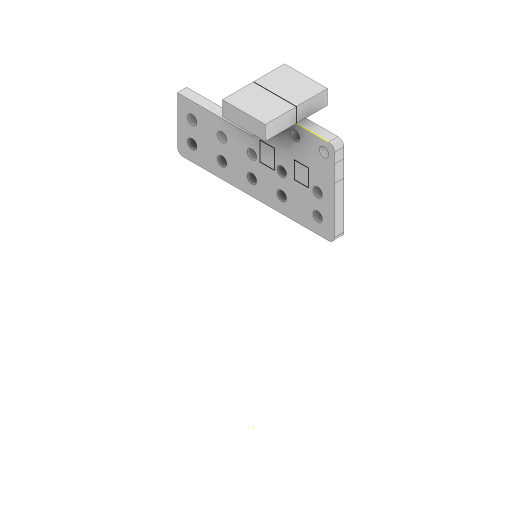
# Autodesk Inventor part: upper diod hplder
Saved by Autodesk Inventor 2023.2 (Build 272271000, 271)
## iProperties
Created: 2023-04-12
Part Number: upper diod hplder
Material: Типовые
Document SubType Name: Modeling
Designer: User
Density: 1 g/cm^3
Appearance: По умолчанию
Author: User
Autodesk Inventor part; units mm, degrees
(part 1 of 6)
ref_plane "YZ Plane" through (0, 0, 0) normal (1, 0, 0) x (0, 1, 0)
ref_plane "XZ Plane" through (0, 0, 0) normal (0, 1, 0) x (-1, 0, 0)
ref_plane "XY Plane" through (0, 0, 0) normal (0, 0, 1) x (1, 0, 0)
sketch "Эскиз1" plane through (0, 0, 0) normal (0, 0, 1) x (1, 0, 0)
  line L0 (-26.3398, -17.2609) -> (28.1261, -17.2901)
  arc A0 (28.1261, -17.2901) -> (29.0872, -16.3296) centre (28.1266, -16.3296) ccw
  line L1 (29.0872, -16.3296) -> (29.0872, 55.0102)
  arc A1 (29.0872, 55.0102) -> (28.1266, 55.9707) centre (28.1266, 55.0102) ccw
  line L2 (28.1266, 55.9707) -> (-6.6805, 55.9707)
  line L3 (-6.6805, 55.9707) -> (-6.6805, 56.9313)
  line L4 (-6.6805, 56.9313) -> (28.1266, 56.9313)
  arc A2 (30.0477, 55.0102) -> (28.1266, 56.9313) centre (28.1266, 55.0102) ccw
  line L5 (30.0477, 55.0102) -> (30.0477, -16.3296)
  arc A3 (28.1256, -18.2506) -> (30.0477, -16.3296) centre (28.1266, -16.3296) ccw
  line L6 (28.1256, -18.2506) -> (-26.3547, -18.2215)
  arc A4 (-28.2747, -16.2994) -> (-26.3547, -18.2215) centre (-26.3537, -16.3004) ccw
  line L7 (-28.2747, -16.2994) -> (-28.2581, 14.7062)
  line L8 (-28.2581, 14.7062) -> (-28.2581, 55.0102)
  arc A5 (-26.3371, 56.9313) -> (-28.2581, 55.0102) centre (-26.3371, 55.0102) ccw
  line L9 (-26.3371, 56.9313) -> (-24.7345, 56.9313)
  line L10 (-24.7345, 56.9313) -> (-24.7345, 55.9729)
  line L11 (-24.7345, 55.9729) -> (-26.3371, 55.9729)
  arc A6 (-26.3371, 55.9729) -> (-27.2998, 55.0102) centre (-26.3371, 55.0102) ccw
  line L12 (-27.2998, 55.0102) -> (-27.2998, -16.3004)
  arc A7 (-27.2998, -16.3004) -> (-26.3398, -17.2609) centre (-26.3393, -16.3004) ccw
  line L13 (-24.4159, 86.3863) -> (-24.4159, 89.6301)
  arc A8 (-22.4948, 91.5512) -> (-24.4159, 89.6301) centre (-22.4948, 89.6301) ccw
  line L14 (-22.4948, 91.5512) -> (24.2451, 91.5512)
  arc A9 (26.1661, 89.6301) -> (24.2451, 91.5512) centre (24.2451, 89.6301) ccw
  line L15 (26.1661, 89.6301) -> (26.1661, 86.3863)
  arc A10 (-24.4154, 65.9583) -> (-22.4943, 64.0372) centre (-22.4943, 65.9583) ccw
  line L16 (-24.4154, 65.9583) -> (-24.4154, 80.9805)
  line L17 (26.1662, 80.9805) -> (26.1662, 65.9583)
  arc A11 (24.2452, 64.0372) -> (26.1662, 65.9583) centre (24.2452, 65.9583) ccw
  line L18 (24.2452, 64.0372) -> (-22.4943, 64.0372)
  line L19 (22.2378, -70.3584) -> (22.2378, -67.7272)
  line L20 (22.2378, -67.7272) -> (21.6859, -67.7272)
  line L21 (21.6859, -67.7272) -> (20.7902, -70.4344)
  line L22 (8.3577, -67.7272) -> (7.4019, -67.7272)
  line L23 (7.4019, -67.7272) -> (7.4019, -70.3584)
  line L24 (5.4825, -69.6386) -> (5.4825, -67.7272)
  line L25 (5.4825, -67.7272) -> (4.5267, -67.7272)
  line L26 (-5.5224, -67.4872) -> (-5.5224, -68.6829)
  line L27 (-5.5224, -68.6829) -> (-4.0908, -68.6829)
  line L28 (-4.0908, -68.6829) -> (-4.0908, -67.4872)
  line L29 (-4.0908, -70.3584) -> (-4.0908, -69.1628)
  line L30 (-4.0908, -69.1628) -> (-5.5224, -69.1628)
  line L31 (-5.5224, -69.1628) -> (-5.5224, -70.3584)
  line L32 (-15.6236, -67.4872) -> (-15.6236, -68.8988)
  line L33 (-15.6236, -68.8988) -> (-14.104, -67.3033)
  line L34 (-13.7881, -67.6672) -> (-14.7518, -68.6789)
  line L35 (-14.7518, -68.6789) -> (-13.7641, -70.2025)
  line L36 (-17.4951, -69.6386) -> (-17.4951, -67.7272)
  line L37 (-17.4951, -67.7272) -> (-18.4508, -67.7272)
  line L38 (-11.6305, -61.3315) -> (-12.5526, -59.9509)
  line L39 (-12.5526, -59.9509) -> (-13.4746, -61.3315)
  line L40 (-13.9674, -61.0047) -> (-12.9087, -59.4191)
  line L41 (-12.9087, -59.4191) -> (-13.9674, -57.8336)
  line L42 (-13.4746, -57.5067) -> (-12.5526, -58.8873)
  line L43 (-12.5526, -58.8873) -> (-11.6305, -57.5067)
  line L44 (-11.1378, -57.8336) -> (-12.1964, -59.4191)
  line L45 (-12.1964, -59.4191) -> (-11.1378, -61.0047)
  line L46 (-23.4868, -54.0669) -> (-21.5482, -59.7997)
  line L47 (-21.5482, -59.7997) -> (-19.6095, -54.0669)
  line L48 (16.563, -44.8841) -> (17.5187, -44.8841)
  line L49 (17.5187, -44.8841) -> (17.5187, -43.9283)
  line L50 (17.5187, -43.9283) -> (16.563, -43.9283)
  line L51 (17.5187, -46.5596) -> (17.5187, -45.3639)
  line L52 (17.5187, -45.3639) -> (16.9309, -45.3639)
  line L53 (16.9309, -45.3639) -> (16.0471, -46.6916)
  line L54 (14.1677, -45.8398) -> (14.1677, -43.9283)
  line L55 (14.1677, -43.9283) -> (13.2119, -43.9283)
  line L56 (-1.152, -46.5596) -> (-1.152, -43.9283)
  line L57 (-1.152, -43.9283) -> (-1.7039, -43.9283)
  line L58 (-1.7039, -43.9283) -> (-2.5996, -46.6356)
  line L59 (-15.0321, -43.9283) -> (-15.9878, -43.9283)
  line L60 (-15.9878, -43.9283) -> (-15.9878, -46.5596)
  line L61 (-17.9073, -45.8398) -> (-17.9073, -43.9283)
  line L62 (-17.9073, -43.9283) -> (-18.863, -43.9283)
  line L63 (23.6577, -19.6659) -> (22.7019, -19.6659)
  line L64 (22.7019, -19.6659) -> (22.7019, -22.0572)
  line L65 (22.7019, -22.0572) -> (23.6577, -22.0572)
  line L66 (23.6577, -22.5371) -> (22.7019, -22.5371)
  line L67 (22.7019, -22.5371) -> (22.7019, -23.7327)
  line L68 (19.3509, -20.1418) -> (19.3509, -20.6216)
  line L69 (19.3509, -20.6216) -> (20.7825, -20.6216)
  line L70 (20.7825, -20.6216) -> (20.7825, -20.1418)
  line L71 (21.0224, -21.1015) -> (19.3509, -21.1015)
  line L72 (19.3509, -21.1015) -> (19.3509, -21.5773)
  line L73 (-20.9709, -32.5834) -> (-20.9709, -36.6502)
  line L74 (-20.9709, -36.6502) -> (-19.2954, -36.6502)
  line L75 (-7.2481, -21.1565) -> (-8.2038, -21.1565)
  line L76 (-8.2038, -21.1565) -> (-8.2038, -22.1122)
  line L77 (-8.2038, -22.1122) -> (-7.2481, -22.1122)
  line L78 (-8.2038, -19.4809) -> (-8.2038, -20.6766)
  line L79 (-8.2038, -20.6766) -> (-7.2481, -20.6766)
  line L80 (-13.9502, -22.1122) -> (-12.9945, -22.1122)
  line L81 (-12.9945, -22.1122) -> (-12.9945, -19.4809)
  line L82 (9.9855, -5.8573) -> (9.0298, -5.8573)
  line L83 (9.0298, -5.8573) -> (9.0298, -8.4886)
  line L84 (7.1103, -7.7688) -> (7.1103, -5.8573)
  line L85 (7.1103, -5.8573) -> (6.1546, -5.8573)
  line L86 (7.8829, 3.9338) -> (6.9272, 3.9338)
  line L87 (6.9272, 3.9338) -> (6.9272, 1.3026)
  line L88 (-12.8449, -8.5847) -> (-12.8449, -7.629)
  line L89 (-12.8449, -7.629) -> (-14.2805, -7.629)
  line L90 (-14.2765, -7.1491) -> (-12.8449, -7.1491)
  line L91 (-12.8449, -7.1491) -> (-12.8449, -4.9978)
  line L92 (-19.7789, -5.2377) -> (-21.4584, -5.2377)
  line L93 (-21.4584, -5.2377) -> (-21.4584, -6.6733)
  line L94 (-21.4584, -6.6733) -> (-20.2548, -6.6733)
  line L95 (-20.2548, -7.1531) -> (-21.4584, -7.1531)
  line L96 (-21.4584, -7.1531) -> (-21.4584, -9.0646)
  line L97 (-21.4584, -9.0646) -> (-19.7789, -9.0646)
  line L98 (-10.2251, 3.7997) -> (-11.1809, 3.7997)
  line L99 (-11.1809, 3.7997) -> (-11.1809, 1.4084)
  line L100 (-11.1809, 1.4084) -> (-10.2251, 1.4084)
  line L101 (-10.2251, 0.9285) -> (-11.1809, 0.9285)
  line L102 (-11.1809, 0.9285) -> (-11.1809, -0.2671)
  line L103 (-21.234, 4.0396) -> (-21.234, 2.844)
  line L104 (-21.234, 2.844) -> (-19.8024, 2.844)
  line L105 (-19.8024, 2.844) -> (-19.8024, 4.0396)
  line L106 (-19.8024, 1.1685) -> (-19.8024, 2.3641)
  line L107 (-19.8024, 2.3641) -> (-21.234, 2.3641)
  line L108 (-21.234, 2.3641) -> (-21.234, 1.1685)
  line L109 (-22.0384, 40.4901) -> (-22.0384, 38.1581)
  line L110 (-22.0384, 42.8269) -> (-22.0384, 41.0755)
  line L111 (14.204, 105.6579) -> (17.5277, 105.6579)
  line L112 (17.5277, 105.6579) -> (17.5277, 100.6124)
  line L113 (17.5277, 100.6124) -> (16.6777, 100.6124)
  line L114 (16.6777, 100.6124) -> (16.6777, 104.9441)
  line L115 (16.6777, 104.9441) -> (14.945, 104.9441)
  line L116 (13.0761, 100.6124) -> (13.0761, 101.3534)
  line L117 (13.0761, 101.3534) -> (13.1197, 101.3534)
  line L118 (4.3473, 100.8685) -> (4.3473, 98.7544)
  line L119 (4.3473, 98.7544) -> (3.4973, 98.7544)
  line L120 (3.4973, 98.7544) -> (3.4973, 105.6579)
  line L121 (3.4973, 105.6579) -> (4.3473, 105.6579)
  line L122 (4.3473, 105.6579) -> (4.3473, 105.1294)
  line L123 (-2.894, 100.6124) -> (-2.894, 102.8845)
  line L124 (-2.894, 102.8845) -> (-5.1716, 102.8845)
  line L125 (-5.1716, 102.8845) -> (-5.1716, 100.6124)
  line L126 (-5.1716, 100.6124) -> (-6.0216, 100.6124)
  line L127 (-6.0216, 100.6124) -> (-6.0216, 105.6579)
  line L128 (-6.0216, 105.6579) -> (-5.1716, 105.6579)
  line L129 (-5.1716, 105.6579) -> (-5.1716, 103.6146)
  line L130 (-5.1716, 103.6146) -> (-2.894, 103.6146)
  line L131 (-2.894, 103.6146) -> (-2.894, 105.6579)
  line L132 (-2.894, 105.6579) -> (-2.044, 105.6579)
  line L133 (-2.044, 105.6579) -> (-2.044, 100.6124)
  line L134 (-2.044, 100.6124) -> (-2.894, 100.6124)
  line L135 (-1.8953, 95.9463) -> (-2.3751, 95.9463)
  line L136 (-2.3751, 95.9463) -> (-2.3751, 94.9906)
  line L137 (-2.3751, 94.9906) -> (-1.8953, 94.9906)
  line L138 (-2.3751, 97.6218) -> (-2.3751, 96.4262)
  line L139 (-2.3751, 96.4262) -> (-1.8953, 96.4262)
  line L140 (-12.9122, 94.7506) -> (-12.9122, 97.3819)
  line L141 (-12.9122, 97.3819) -> (-13.8679, 97.3819)
  line L142 (-13.8679, 97.3819) -> (-13.8679, 94.7506)
  line L143 (-11.9524, 97.3819) -> (-12.4323, 97.3819)
  line L144 (-12.4323, 97.3819) -> (-12.4323, 94.7506)
  line L145 (-19.6143, 94.9906) -> (-18.6586, 94.9906)
  line L146 (-18.6586, 94.9906) -> (-18.6586, 97.6218)
  arc A12 (-26.3365, -20.5722) -> (-28.2575, -22.4932) centre (-26.3365, -22.4932) ccw
  line L147 (-26.3365, -20.5722) -> (-24.7339, -20.5722)
  line L148 (-24.7339, -20.5722) -> (-24.7339, -21.5327)
  line L149 (-24.7339, -21.5327) -> (-26.3365, -21.5327)
  arc A13 (-26.3365, -21.5327) -> (-27.297, -22.4932) centre (-26.3365, -22.4932) ccw
  line L150 (-27.297, -22.4932) -> (-27.297, -37.7101)
  arc A14 (-27.297, -37.7101) -> (-26.3365, -38.6706) centre (-26.3365, -37.7101) ccw
  line L151 (-26.3365, -38.6706) -> (-0.1998, -38.6706)
  arc A15 (-0.1998, -38.6706) -> (0.7607, -37.7101) centre (-0.1998, -37.7101) ccw
  line L152 (0.7607, -37.7101) -> (0.7607, -22.4932)
  arc A16 (0.7607, -22.4932) -> (-0.1998, -21.5327) centre (-0.1998, -22.4932) ccw
  line L153 (-0.1998, -21.5327) -> (-3.2963, -21.5327)
  line L154 (-3.2963, -21.5327) -> (-3.2963, -20.5722)
  line L155 (-3.2963, -20.5722) -> (-0.1998, -20.5722)
  arc A17 (1.7212, -22.4932) -> (-0.1998, -20.5722) centre (-0.1998, -22.4932) ccw
  line L156 (1.7212, -22.4932) -> (1.7212, -37.7101)
  arc A18 (-0.1998, -39.6312) -> (1.7212, -37.7101) centre (-0.1998, -37.7101) ccw
  line L157 (-0.1998, -39.6312) -> (-26.3365, -39.6312)
  arc A19 (-28.2575, -37.7101) -> (-26.3365, -39.6312) centre (-26.3365, -37.7101) ccw
  line L158 (-28.2575, -37.7101) -> (-28.2575, -22.4932)
  line L159 (6.4559, -20.5722) -> (6.4559, -21.5327)
  line L160 (6.4559, -21.5327) -> (5.6511, -21.5327)
  arc A20 (5.6511, -21.5327) -> (4.6905, -22.4932) centre (5.6511, -22.4932) ccw
  line L161 (4.6905, -22.4932) -> (4.6905, -37.7101)
  arc A21 (4.6905, -37.7101) -> (5.6511, -38.6706) centre (5.6511, -37.7101) ccw
  line L162 (5.6511, -38.6706) -> (28.0873, -38.6706)
  arc A22 (28.0873, -38.6706) -> (29.0478, -37.7101) centre (28.0873, -37.7101) ccw
  line L163 (29.0478, -37.7101) -> (29.0478, -22.4932)
  arc A23 (29.0478, -22.4932) -> (28.0873, -21.5327) centre (28.0873, -22.4932) ccw
  line L164 (28.0873, -21.5327) -> (26.8887, -21.5327)
  line L165 (26.8887, -21.5327) -> (26.8887, -20.5722)
  line L166 (26.8887, -20.5722) -> (28.0873, -20.5722)
  arc A24 (30.0083, -22.4932) -> (28.0873, -20.5722) centre (28.0873, -22.4932) ccw
  line L167 (30.0083, -22.4932) -> (30.0083, -37.7101)
  arc A25 (28.0873, -39.6312) -> (30.0083, -37.7101) centre (28.0873, -37.7101) ccw
  line L168 (28.0873, -39.6312) -> (5.6511, -39.6312)
  arc A26 (3.73, -37.7101) -> (5.6511, -39.6312) centre (5.6511, -37.7101) ccw
  line L169 (3.73, -37.7101) -> (3.73, -22.4932)
  arc A27 (5.6511, -20.5722) -> (3.73, -22.4932) centre (5.6511, -22.4932) ccw
  line L170 (5.6511, -20.5722) -> (6.4559, -20.5722)
  arc A28 (-26.4304, -44.783) -> (-28.3515, -46.704) centre (-26.4304, -46.704) ccw
  line L171 (-26.4304, -44.783) -> (-24.7339, -44.783)
  line L172 (-24.7339, -44.783) -> (-24.7339, -45.7435)
  line L173 (-24.7339, -45.7435) -> (-26.4304, -45.7435)
  arc A29 (-26.4304, -45.7435) -> (-27.391, -46.704) centre (-26.4304, -46.704) ccw
  line L174 (-27.391, -46.704) -> (-27.391, -95.6666)
  arc A30 (-27.391, -95.6666) -> (-26.4304, -96.6271) centre (-26.4304, -95.6666) ccw
  line L175 (-26.4304, -96.6271) -> (27.8395, -96.6271)
  arc A31 (27.8395, -96.6271) -> (28.8, -95.6666) centre (27.8395, -95.6666) ccw
  line L176 (28.8, -95.6666) -> (28.8, -46.704)
  arc A32 (28.8, -46.704) -> (27.8395, -45.7435) centre (27.8395, -46.704) ccw
  line L177 (27.8395, -45.7435) -> (19.8909, -45.7435)
  line L178 (19.8909, -45.7435) -> (19.8909, -44.783)
  line L179 (19.8909, -44.783) -> (27.8395, -44.783)
  arc A33 (29.7605, -46.704) -> (27.8395, -44.783) centre (27.8395, -46.704) ccw
  line L180 (29.7605, -46.704) -> (29.7605, -95.6666)
  arc A34 (27.8395, -97.5877) -> (29.7605, -95.6666) centre (27.8395, -95.6666) ccw
  line L181 (27.8395, -97.5877) -> (-26.4304, -97.5877)
  arc A35 (-28.3515, -95.6666) -> (-26.4304, -97.5877) centre (-26.4304, -95.6666) ccw
  line L182 (-28.3515, -95.6666) -> (-28.3515, -46.704)
  line L183 (-9.5571, 96.906) -> (-9.5571, 96.4262)
  line L184 (-9.5571, 96.4262) -> (-8.1255, 96.4262)
  line L185 (-8.1255, 96.4262) -> (-8.1255, 96.906)
  line L186 (-7.8856, 95.9463) -> (-9.5571, 95.9463)
  line L187 (-9.5571, 95.9463) -> (-9.5571, 95.4704)
  line L188 (-4.2946, 94.7506) -> (-4.2946, 96.878)
  line L189 (-4.2946, 96.878) -> (-5.0544, 95.8103)
  line L190 (-5.4463, 95.8103) -> (-6.2061, 96.878)
  line L191 (-6.2061, 96.878) -> (-6.2061, 94.7506)
  line L192 (-6.25, 97.7618) -> (-5.2503, 96.3582)
  line L193 (-5.2503, 96.3582) -> (-4.2506, 97.7618)
  line L194 (-13.6389, 103.2931) -> (-11.5902, 100.6124)
  line L195 (-11.5902, 100.6124) -> (-12.6472, 100.6124)
  line L196 (-12.6472, 100.6124) -> (-14.3745, 102.939)
  line L197 (-14.3745, 102.939) -> (-14.794, 102.939)
  line L198 (-14.794, 102.939) -> (-14.794, 100.6124)
  line L199 (-14.794, 100.6124) -> (-15.644, 100.6124)
  line L200 (-15.644, 100.6124) -> (-15.644, 105.6579)
  line L201 (-15.644, 105.6579) -> (-14.794, 105.6579)
  line L202 (-14.794, 105.6579) -> (-14.794, 103.4621)
  line L203 (-12.1677, 105.6579) -> (-11.9389, 105.6579)
  line L204 (-11.9389, 105.6579) -> (-11.9389, 104.9278)
  line L205 (-11.9389, 104.9278) -> (-12.135, 104.9278)
  line L206 (1.1489, 104.9169) -> (1.1489, 100.6124)
  line L207 (1.1489, 100.6124) -> (0.2989, 100.6124)
  line L208 (0.2989, 100.6124) -> (0.2989, 104.9169)
  line L209 (0.2989, 104.9169) -> (-1.4174, 104.9169)
  line L210 (-1.4174, 104.9169) -> (-1.4174, 105.6579)
  line L211 (-1.4174, 105.6579) -> (2.8653, 105.6579)
  line L212 (2.8653, 105.6579) -> (2.8653, 104.9169)
  line L213 (2.8653, 104.9169) -> (1.1489, 104.9169)
  line L214 (20.2412, 103.0044) -> (19.6091, 103.0044)
  line L215 (19.6091, 103.0044) -> (19.6091, 101.288)
  line L216 (19.6091, 101.288) -> (20.2194, 101.288)
  line L217 (20.5245, 100.6124) -> (18.7591, 100.6124)
  line L218 (18.7591, 100.6124) -> (18.7591, 105.6579)
  line L219 (18.7591, 105.6579) -> (19.6091, 105.6579)
  line L220 (19.6091, 105.6579) -> (19.6091, 103.6909)
  line L221 (19.6091, 103.6909) -> (20.5463, 103.6909)
  line L222 (-19.4405, 52.5558) -> (-20.3962, 52.5558)
  line L223 (-2.3684, 29.0322) -> (-3.0595, 29.0322)
  line L224 (-3.0595, 29.0322) -> (-3.0595, 28.1573)
  line L225 (17.7134, 28.6956) -> (17.7134, 29.0126)
  line L226 (17.7134, 29.0126) -> (17.0223, 29.0126)
  line L227 (-16.4514, 1.8882) -> (-16.4514, 3.7997)
  line L228 (-16.4514, 3.7997) -> (-17.4071, 3.7997)
  line L229 (-13.5762, 3.7997) -> (-14.5319, 3.7997)
  line L230 (-14.5319, 3.7997) -> (-14.5319, 1.1685)
  line L231 (-15.3154, 7.3282) -> (-16.719, 9.8275)
  line L232 (-16.719, 9.8275) -> (-17.2869, 9.2676)
  line L233 (-17.2869, 9.2676) -> (-17.2869, 7.4441)
  line L234 (-17.2869, 11.7509) -> (-17.2869, 9.9194)
  line L235 (-17.2869, 9.9194) -> (-15.2714, 11.9189)
  line L236 (-14.9355, 11.583) -> (-16.3631, 10.1634)
  line L237 (-16.3631, 10.1634) -> (-14.8915, 7.5601)
  line L238 (-9.014, -9.3045) -> (-9.014, -5.2377)
  line L239 (-9.014, -5.2377) -> (-10.9254, -5.2377)
  line L240 (-10.9254, -5.2377) -> (-10.9254, -9.3045)
  line L241 (11.7098, 2.0224) -> (11.7098, 3.9338)
  line L242 (11.7098, 3.9338) -> (10.7541, 3.9338)
  line L243 (14.585, 3.9338) -> (13.6293, 3.9338)
  line L244 (13.6293, 3.9338) -> (13.6293, 1.5425)
  line L245 (13.6293, 1.5425) -> (14.585, 1.5425)
  line L246 (14.585, 1.0626) -> (13.6293, 1.0626)
  line L247 (13.6293, 1.0626) -> (13.6293, -0.133)
  line L248 (13.8124, -7.7688) -> (13.8124, -5.8573)
  line L249 (13.8124, -5.8573) -> (12.8567, -5.8573)
  line L250 (17.1635, -8.4886) -> (17.1635, -5.8573)
  line L251 (17.1635, -5.8573) -> (16.6117, -5.8573)
  line L252 (16.6117, -5.8573) -> (15.7159, -8.5646)
  line L253 (-19.6966, -21.6323) -> (-19.6966, -19.7209)
  line L254 (-19.6966, -19.7209) -> (-20.6523, -19.7209)
  line L255 (-16.8214, -19.7209) -> (-17.7771, -19.7209)
  line L256 (-17.7771, -19.7209) -> (-17.7771, -22.3521)
  line L257 (-20.1571, -26.5082) -> (-21.3527, -26.5082)
  line L258 (-21.3527, -26.5082) -> (-21.3527, -30.3351)
  line L259 (-21.3527, -30.3351) -> (-20.1571, -30.3351)
  line L260 (-22.6464, -32.8233) -> (-24.322, -32.8233)
  line L261 (-24.322, -32.8233) -> (-24.322, -34.2509)
  line L262 (-24.322, -34.2509) -> (-22.6464, -34.2509)
  line L263 (-22.6464, -34.7308) -> (-24.322, -34.7308)
  line L264 (-24.322, -34.7308) -> (-24.322, -36.8902)
  line L265 (9.5336, -22.0572) -> (10.4894, -22.0572)
  line L266 (10.4894, -22.0572) -> (10.4894, -19.426)
  line L267 (17.4314, -22.2971) -> (17.4314, -20.1697)
  line L268 (17.4314, -20.1697) -> (16.6716, -21.2374)
  line L269 (16.2797, -21.2374) -> (15.52, -20.1697)
  line L270 (15.52, -20.1697) -> (15.52, -22.2971)
  line L271 (15.476, -19.286) -> (16.4757, -20.6896)
  line L272 (16.4757, -20.6896) -> (17.4754, -19.286)
  line L273 (7.2453, -25.0001) -> (7.4333, -25.0001)
  line L274 (7.4333, -25.0001) -> (6.3616, -23.9764)
  line L275 (8.441, -24.0444) -> (7.1254, -24.0444)
  line L276 (7.1254, -24.0444) -> (8.393, -25.256)
  line L277 (11.5521, -27.3914) -> (11.5521, -25.48)
  line L278 (11.5521, -25.48) -> (10.5964, -25.48)
  line L279 (14.4273, -25.48) -> (13.4716, -25.48)
  line L280 (13.4716, -25.48) -> (13.4716, -27.8713)
  line L281 (13.4716, -27.8713) -> (14.4273, -27.8713)
  line L282 (14.4273, -28.3512) -> (13.4716, -28.3512)
  line L283 (13.4716, -28.3512) -> (13.4716, -29.5468)
  line L284 (8.138, -34.5782) -> (8.138, -32.6667)
  line L285 (8.138, -32.6667) -> (7.1823, -32.6667)
  line L286 (10.0095, -32.4268) -> (10.0095, -33.8384)
  line L287 (10.0095, -33.8384) -> (11.5291, -32.2428)
  line L288 (11.845, -32.6067) -> (10.8812, -33.6184)
  line L289 (10.8812, -33.6184) -> (11.869, -35.142)
  line L290 (-22.6899, -43.6884) -> (-22.6899, -44.8841)
  line L291 (-22.6899, -44.8841) -> (-21.2583, -44.8841)
  line L292 (-21.2583, -44.8841) -> (-21.2583, -43.6884)
  line L293 (-21.2583, -46.5596) -> (-21.2583, -45.3639)
  line L294 (-21.2583, -45.3639) -> (-22.6899, -45.3639)
  line L295 (-22.6899, -45.3639) -> (-22.6899, -46.5596)
  line L296 (-11.681, -43.9283) -> (-12.6368, -43.9283)
  line L297 (-12.6368, -43.9283) -> (-12.6368, -46.3197)
  line L298 (-12.6368, -46.3197) -> (-11.681, -46.3197)
  line L299 (-11.681, -46.7995) -> (-12.6368, -46.7995)
  line L300 (-12.6368, -46.7995) -> (-12.6368, -47.9952)
  line L301 (-7.8541, -45.8398) -> (-7.8541, -43.9283)
  line L302 (-7.8541, -43.9283) -> (-8.8099, -43.9283)
  line L303 (1.2433, -44.8841) -> (2.199, -44.8841)
  line L304 (2.199, -44.8841) -> (2.199, -43.9283)
  line L305 (2.199, -43.9283) -> (1.2433, -43.9283)
  line L306 (2.199, -46.5596) -> (2.199, -45.3639)
  line L307 (2.199, -45.3639) -> (1.6112, -45.3639)
  line L308 (1.6112, -45.3639) -> (0.7275, -46.6916)
  line L309 (4.1185, -43.6884) -> (4.1185, -44.8841)
  line L310 (4.1185, -44.8841) -> (4.5944, -44.8841)
  line L311 (4.5944, -44.8841) -> (4.5944, -44.2602)
  line L312 (4.5944, -45.9878) -> (4.5944, -45.3639)
  line L313 (4.5944, -45.3639) -> (4.1185, -45.3639)
  line L314 (4.1185, -45.3639) -> (4.1185, -46.5596)
  line L315 (9.385, -43.6884) -> (9.385, -46.3197)
  line L316 (9.385, -46.3197) -> (10.3408, -46.3197)
  line L317 (10.3408, -46.3197) -> (10.3408, -43.6884)
  line L318 (10.8206, -43.6884) -> (10.8206, -46.3197)
  line L319 (10.8206, -46.3197) -> (11.0606, -46.3197)
  line L320 (10.8206, -47.0355) -> (10.8206, -46.7995)
  line L321 (10.8206, -46.7995) -> (8.4253, -46.7995)
  line L322 (8.4293, -46.3197) -> (8.9052, -46.3197)
  line L323 (8.9052, -46.3197) -> (8.9052, -43.6884)
  line L324 (-22.2777, -67.4872) -> (-22.2777, -68.6829)
  line L325 (-22.2777, -68.6829) -> (-20.8461, -68.6829)
  line L326 (-20.8461, -68.6829) -> (-20.8461, -67.4872)
  line L327 (-20.8461, -70.3584) -> (-20.8461, -69.1628)
  line L328 (-20.8461, -69.1628) -> (-22.2777, -69.1628)
  line L329 (-22.2777, -69.1628) -> (-22.2777, -70.3584)
  line L330 (-10.7929, -70.3584) -> (-10.7929, -67.7272)
  line L331 (-10.7929, -67.7272) -> (-11.3448, -67.7272)
  line L332 (-11.3448, -67.7272) -> (-12.2405, -70.4344)
  line L333 (0.6998, -67.4872) -> (0.6998, -68.6829)
  line L334 (0.6998, -68.6829) -> (2.1314, -68.6829)
  line L335 (2.1314, -68.6829) -> (2.1314, -67.4872)
  line L336 (2.1314, -70.3584) -> (2.1314, -69.1628)
  line L337 (2.1314, -69.1628) -> (0.6998, -69.1628)
  line L338 (0.6998, -69.1628) -> (0.6998, -70.3584)
  line L339 (11.7087, -67.7272) -> (10.753, -67.7272)
  line L340 (10.753, -67.7272) -> (10.753, -70.1185)
  line L341 (10.753, -70.1185) -> (11.7087, -70.1185)
  line L342 (11.7087, -70.5983) -> (10.753, -70.5983)
  line L343 (10.753, -70.5983) -> (10.753, -71.794)
  line L344 (15.5356, -69.6386) -> (15.5356, -67.7272)
  line L345 (15.5356, -67.7272) -> (14.5799, -67.7272)
  arc A36 (-26.3371, 96.7637) -> (-28.2581, 94.8427) centre (-26.3371, 94.8427) ccw
  line L346 (-26.3371, 96.7637) -> (-24.7345, 96.7637)
  line L347 (-24.7345, 96.7637) -> (-24.7345, 95.803)
  line L348 (-24.7345, 95.803) -> (-26.3371, 95.803)
  arc A37 (-26.3371, 95.803) -> (-27.2974, 94.8427) centre (-26.3371, 94.8427) ccw
  line L349 (-27.2974, 94.8427) -> (-27.2974, 63.0544)
  arc A38 (-27.2974, 63.0544) -> (-26.3371, 62.0941) centre (-26.3371, 63.0544) ccw
  line L350 (-26.3371, 62.0941) -> (28.0873, 62.0941)
  arc A39 (28.0873, 62.0941) -> (29.0477, 63.0544) centre (28.0873, 63.0544) ccw
  line L351 (29.0477, 63.0544) -> (29.0477, 94.8427)
  arc A40 (29.0477, 94.8427) -> (28.0873, 95.803) centre (28.0873, 94.8427) ccw
  line L352 (28.0873, 95.803) -> (1.4111, 95.803)
  line L353 (1.4111, 95.803) -> (1.4111, 96.7637)
  line L354 (1.4111, 96.7637) -> (28.0873, 96.7637)
  arc A41 (30.0084, 94.8427) -> (28.0873, 96.7637) centre (28.0873, 94.8427) ccw
  line L355 (30.0084, 94.8427) -> (30.0084, 63.0544)
  arc A42 (28.0873, 61.1334) -> (30.0084, 63.0544) centre (28.0873, 63.0544) ccw
  line L356 (28.0873, 61.1334) -> (-26.3371, 61.1334)
  arc A43 (-28.2581, 63.0544) -> (-26.3371, 61.1334) centre (-26.3371, 63.0544) ccw
  line L357 (-28.2581, 63.0544) -> (-28.2581, 94.8427)
  arc A44 (-23.4577, 51.5612) -> (-25.3787, 49.6401) centre (-23.4577, 49.6401) ccw
  line L358 (-23.4577, 51.5612) -> (-22.722, 51.5612)
  line L359 (-22.722, 51.5612) -> (-22.722, 50.5909)
  line L360 (-22.722, 50.5909) -> (-23.4577, 50.5909)
  arc A45 (-23.4577, 50.5909) -> (-24.4084, 49.6401) centre (-23.4577, 49.6401) ccw
  line L361 (-24.4084, 49.6401) -> (-24.4084, 15.3591)
  arc A46 (-24.4084, 15.3591) -> (-23.4577, 14.4084) centre (-23.4577, 15.3591) ccw
  line L362 (-23.4577, 14.4084) -> (25.245, 14.4084)
  arc A47 (25.245, 14.4084) -> (26.1958, 15.3591) centre (25.245, 15.3591) ccw
  line L363 (26.1958, 15.3591) -> (26.1958, 49.6401)
  arc A48 (26.1958, 49.6401) -> (25.245, 50.5909) centre (25.245, 49.6401) ccw
  line L364 (25.245, 50.5909) -> (-12.6469, 50.5909)
  line L365 (-12.6469, 50.5909) -> (-12.6469, 51.5612)
  line L366 (-12.6469, 51.5612) -> (25.245, 51.5612)
  arc A49 (27.1661, 49.6401) -> (25.245, 51.5612) centre (25.245, 49.6401) ccw
  line L367 (27.1661, 49.6401) -> (27.1661, 15.3591)
  arc A50 (25.245, 13.4381) -> (27.1661, 15.3591) centre (25.245, 15.3591) ccw
  line L368 (25.245, 13.4381) -> (-23.4577, 13.4381)
  arc A51 (-25.3787, 15.3591) -> (-23.4577, 13.4381) centre (-23.4577, 15.3591) ccw
  line L369 (-25.3787, 15.3591) -> (-25.3787, 49.6401)
  line L370 (-22.6498, 10.3178) -> (-22.6498, 9.3573)
  line L371 (-22.6498, 9.3573) -> (-23.4549, 9.3573)
  arc A52 (-23.4549, 9.3573) -> (-24.4154, 8.3967) centre (-23.4549, 8.3967) ccw
  line L372 (-24.4154, 8.3967) -> (-24.4154, -13.6995)
  arc A53 (-24.4154, -13.6995) -> (-23.4549, -14.66) centre (-23.4549, -13.6995) ccw
  line L373 (-23.4549, -14.66) -> (25.2057, -14.66)
  arc A54 (25.2057, -14.66) -> (26.1662, -13.6995) centre (25.2057, -13.6995) ccw
  line L374 (26.1662, -13.6995) -> (26.1662, 8.3967)
  arc A55 (26.1662, 8.3967) -> (25.2057, 9.3573) centre (25.2057, 8.3967) ccw
  line L375 (25.2057, 9.3573) -> (-14.1206, 9.3573)
  line L376 (-14.1206, 9.3573) -> (-14.1206, 10.3178)
  line L377 (-14.1206, 10.3178) -> (25.2057, 10.3178)
  arc A56 (27.1267, 8.3967) -> (25.2057, 10.3178) centre (25.2057, 8.3967) ccw
  line L378 (27.1267, 8.3967) -> (27.1267, -13.6995)
  arc A57 (25.2057, -15.6206) -> (27.1267, -13.6995) centre (25.2057, -13.6995) ccw
  line L379 (25.2057, -15.6206) -> (-23.4549, -15.6206)
  arc A58 (-25.3759, -13.6995) -> (-23.4549, -15.6206) centre (-23.4549, -13.6995) ccw
  line L380 (-25.3759, -13.6995) -> (-25.3759, 8.3967)
  arc A59 (-23.4549, 10.3178) -> (-25.3759, 8.3967) centre (-23.4549, 8.3967) ccw
  line L381 (-23.4549, 10.3178) -> (-22.6498, 10.3178)
  line L382 (1.6803, -50.6537) -> (1.6803, -64.5814)
  line L383 (1.6803, -64.5814) -> (23.7725, -64.5814)
  line L384 (23.7725, -64.5814) -> (23.7725, -50.6537)
  line L385 (23.7725, -50.6537) -> (1.6803, -50.6537)
  line L386 (0.2713, 48.7668) -> (0.2713, 34.8391)
  line L387 (0.2713, 34.8391) -> (22.3635, 34.8391)
  line L388 (22.3635, 34.8391) -> (22.3635, 48.7668)
  line L389 (22.3635, 48.7668) -> (0.2713, 48.7668)
  arc A60 (30.7211, -104.1068) -> (33.6027, -101.2252) centre (30.7211, -101.2252) ccw
  line L390 (30.7211, -104.1068) -> (-30.7528, -104.1068)
  arc A61 (-33.6344, -101.2252) -> (-30.7528, -104.1068) centre (-30.7528, -101.2252) ccw
  line L391 (-33.6344, -101.2252) -> (-33.6344, 107.2096)
  arc A62 (-30.7528, 110.0912) -> (-33.6344, 107.2096) centre (-30.7528, 107.2096) ccw
  line L392 (-30.7528, 110.0912) -> (30.7211, 110.0912)
  arc A63 (33.6027, 107.2096) -> (30.7211, 110.0912) centre (30.7211, 107.2096) ccw
  line L393 (33.6027, 107.2096) -> (33.6027, -101.2252)
  spline S0 degree 2 poles (22.4777, -70.5983) (22.2378, -70.5983) (22.2378, -70.3584) knots 0 0 0 1 1 1
  line L394 (22.4777, -70.5983) -> (22.2378, -70.5983) construction
  line L395 (22.2378, -70.5983) -> (22.2378, -70.3584) construction
  spline S1 degree 2 poles (20.7902, -70.4344) (20.7382, -70.5983) (20.5782, -70.5983) knots 0 0 0 1 1 1
  line L396 (20.7902, -70.4344) -> (20.7382, -70.5983) construction
  line L397 (20.7382, -70.5983) -> (20.5782, -70.5983) construction
  spline S2 degree 2 poles (20.5782, -70.5983) (20.3263, -70.5983) (20.3263, -70.3704) knots 0 0 0 1 1 1
  line L398 (20.5782, -70.5983) -> (20.3263, -70.5983) construction
  line L399 (20.3263, -70.5983) -> (20.3263, -70.3704) construction
  spline S3 degree 2 poles (20.3263, -70.3704) (20.3263, -70.3264) (20.3423, -70.2824) knots 0 0 0 1 1 1
  line L400 (20.3263, -70.3704) -> (20.3263, -70.3264) construction
  line L401 (20.3263, -70.3264) -> (20.3423, -70.2824) construction
  line L402 (20.3423, -70.2824) -> (21.29, -67.4112)
  spline S4 degree 2 poles (21.29, -67.4112) (21.342, -67.2473) (21.514, -67.2473) knots 0 0 0 1 1 1
  line L403 (21.29, -67.4112) -> (21.342, -67.2473) construction
  line L404 (21.342, -67.2473) -> (21.514, -67.2473) construction
  line L405 (21.514, -67.2473) -> (22.4777, -67.2473)
  spline S5 degree 2 poles (22.4777, -67.2473) (22.7176, -67.2473) (22.7176, -67.4872) knots 0 0 0 1 1 1
  line L406 (22.4777, -67.2473) -> (22.7176, -67.2473) construction
  line L407 (22.7176, -67.2473) -> (22.7176, -67.4872) construction
  line L408 (22.7176, -67.4872) -> (22.7176, -70.3584)
  spline S6 degree 2 poles (22.7176, -70.3584) (22.7176, -70.5983) (22.4777, -70.5983) knots 0 0 0 1 1 1
  line L409 (22.7176, -70.3584) -> (22.7176, -70.5983) construction
  line L410 (22.7176, -70.5983) -> (22.4777, -70.5983) construction
  spline S7 degree 2 poles (9.0735, -70.5983) (8.8335, -70.5983) (8.8335, -70.3584) knots 0 0 0 1 1 1
  line L411 (9.0735, -70.5983) -> (8.8335, -70.5983) construction
  line L412 (8.8335, -70.5983) -> (8.8335, -70.3584) construction
  line L413 (8.8335, -70.3584) -> (8.8335, -68.207)
  spline S8 degree 2 poles (8.8335, -68.207) (8.8335, -68.0111) (8.5536, -67.7272) (8.3577, -67.7272) knots 0 0 0 1 2 2 2
  line L414 (8.8335, -68.207) -> (8.8335, -68.0111) construction
  line L415 (8.8335, -68.0111) -> (8.5536, -67.7272) construction
  line L416 (8.5536, -67.7272) -> (8.3577, -67.7272) construction
  spline S9 degree 2 poles (7.4019, -70.3584) (7.4019, -70.5983) (7.162, -70.5983) knots 0 0 0 1 1 1
  line L417 (7.4019, -70.3584) -> (7.4019, -70.5983) construction
  line L418 (7.4019, -70.5983) -> (7.162, -70.5983) construction
  spline S10 degree 2 poles (7.162, -70.5983) (6.9221, -70.5983) (6.9221, -70.3584) knots 0 0 0 1 1 1
  line L419 (7.162, -70.5983) -> (6.9221, -70.5983) construction
  line L420 (6.9221, -70.5983) -> (6.9221, -70.3584) construction
  line L421 (6.9221, -70.3584) -> (6.9221, -67.4872)
  spline S11 degree 2 poles (6.9221, -67.4872) (6.9221, -67.2473) (7.162, -67.2473) knots 0 0 0 1 1 1
  line L422 (6.9221, -67.4872) -> (6.9221, -67.2473) construction
  line L423 (6.9221, -67.2473) -> (7.162, -67.2473) construction
  line L424 (7.162, -67.2473) -> (8.3577, -67.2473)
  spline S12 degree 2 poles (8.3577, -67.2473) (8.7536, -67.2473) (9.3134, -67.8071) (9.3134, -68.203) knots 0 0 0 1 2 2 2
  line L425 (8.3577, -67.2473) -> (8.7536, -67.2473) construction
  line L426 (8.7536, -67.2473) -> (9.3134, -67.8071) construction
  line L427 (9.3134, -67.8071) -> (9.3134, -68.203) construction
  line L428 (9.3134, -68.203) -> (9.3134, -70.3584)
  spline S13 degree 2 poles (9.3134, -70.3584) (9.3134, -70.5983) (9.0735, -70.5983) knots 0 0 0 1 1 1
  line L429 (9.3134, -70.3584) -> (9.3134, -70.5983) construction
  line L430 (9.3134, -70.5983) -> (9.0735, -70.5983) construction
  spline S14 degree 2 poles (5.0066, -70.1185) (5.2026, -70.1185) (5.4825, -69.8346) (5.4825, -69.6386) knots 0 0 0 1 2 2 2
  line L431 (5.0066, -70.1185) -> (5.2026, -70.1185) construction
  line L432 (5.2026, -70.1185) -> (5.4825, -69.8346) construction
  line L433 (5.4825, -69.8346) -> (5.4825, -69.6386) construction
  spline S15 degree 2 poles (4.5267, -67.7272) (4.3308, -67.7272) (4.0509, -68.0111) (4.0509, -68.207) knots 0 0 0 1 2 2 2
  line L434 (4.5267, -67.7272) -> (4.3308, -67.7272) construction
  line L435 (4.3308, -67.7272) -> (4.0509, -68.0111) construction
  line L436 (4.0509, -68.0111) -> (4.0509, -68.207) construction
  line L437 (4.0509, -68.207) -> (4.0509, -69.6386)
  spline S16 degree 2 poles (4.0509, -69.6386) (4.0509, -69.8346) (4.3308, -70.1185) (4.5267, -70.1185) knots 0 0 0 1 2 2 2
  line L438 (4.0509, -69.6386) -> (4.0509, -69.8346) construction
  line L439 (4.0509, -69.8346) -> (4.3308, -70.1185) construction
  line L440 (4.3308, -70.1185) -> (4.5267, -70.1185) construction
  line L441 (4.5267, -70.1185) -> (5.0066, -70.1185)
  line L442 (5.0066, -70.5983) -> (4.5267, -70.5983)
  spline S17 degree 2 poles (4.5267, -70.5983) (4.1349, -70.5983) (3.571, -70.0385) (3.571, -69.6426) knots 0 0 0 1 2 2 2
  line L443 (4.5267, -70.5983) -> (4.1349, -70.5983) construction
  line L444 (4.1349, -70.5983) -> (3.571, -70.0385) construction
  line L445 (3.571, -70.0385) -> (3.571, -69.6426) construction
  line L446 (3.571, -69.6426) -> (3.571, -68.203)
  spline S18 degree 2 poles (3.571, -68.203) (3.571, -67.8071) (4.1349, -67.2473) (4.5267, -67.2473) knots 0 0 0 1 2 2 2
  line L447 (3.571, -68.203) -> (3.571, -67.8071) construction
  line L448 (3.571, -67.8071) -> (4.1349, -67.2473) construction
  line L449 (4.1349, -67.2473) -> (4.5267, -67.2473) construction
  line L450 (4.5267, -67.2473) -> (5.7224, -67.2473)
  spline S19 degree 2 poles (5.7224, -67.2473) (5.9623, -67.2473) (5.9623, -67.4872) knots 0 0 0 1 1 1
  line L451 (5.7224, -67.2473) -> (5.9623, -67.2473) construction
  line L452 (5.9623, -67.2473) -> (5.9623, -67.4872) construction
  line L453 (5.9623, -67.4872) -> (5.9623, -69.6346)
  spline S20 degree 2 poles (5.9623, -69.6346) (5.9623, -69.9945) (6.2982, -70.1385) knots 0 0 0 1 1 1
  line L454 (5.9623, -69.6346) -> (5.9623, -69.9945) construction
  line L455 (5.9623, -69.9945) -> (6.2982, -70.1385) construction
  spline S21 degree 2 poles (6.2982, -70.1385) (6.4462, -70.1985) (6.4462, -70.3504) knots 0 0 0 1 1 1
  line L456 (6.2982, -70.1385) -> (6.4462, -70.1985) construction
  line L457 (6.4462, -70.1985) -> (6.4462, -70.3504) construction
  spline S22 degree 2 poles (6.4462, -70.3504) (6.4462, -70.4504) (6.3102, -70.6023) (6.2103, -70.6023) knots 0 0 0 1 2 2 2
  line L458 (6.4462, -70.3504) -> (6.4462, -70.4504) construction
  line L459 (6.4462, -70.4504) -> (6.3102, -70.6023) construction
  line L460 (6.3102, -70.6023) -> (6.2103, -70.6023) construction
  spline S23 degree 2 poles (6.2103, -70.6023) (6.1583, -70.6023) (6.1063, -70.5784) knots 0 0 0 1 1 1
  line L461 (6.2103, -70.6023) -> (6.1583, -70.6023) construction
  line L462 (6.1583, -70.6023) -> (6.1063, -70.5784) construction
  spline S24 degree 2 poles (6.1063, -70.5784) (5.8664, -70.4744) (5.7184, -70.2824) knots 0 0 0 1 1 1
  line L463 (6.1063, -70.5784) -> (5.8664, -70.4744) construction
  line L464 (5.8664, -70.4744) -> (5.7184, -70.2824) construction
  spline S25 degree 2 poles (5.7184, -70.2824) (5.4305, -70.5983) (5.0066, -70.5983) knots 0 0 0 1 1 1
  line L465 (5.7184, -70.2824) -> (5.4305, -70.5983) construction
  line L466 (5.4305, -70.5983) -> (5.0066, -70.5983) construction
  spline S26 degree 2 poles (-4.0908, -67.4872) (-4.0908, -67.2473) (-3.8509, -67.2473) knots 0 0 0 1 1 1
  line L467 (-4.0908, -67.4872) -> (-4.0908, -67.2473) construction
  line L468 (-4.0908, -67.2473) -> (-3.8509, -67.2473) construction
  spline S27 degree 2 poles (-3.8509, -67.2473) (-3.611, -67.2473) (-3.611, -67.4872) knots 0 0 0 1 1 1
  line L469 (-3.8509, -67.2473) -> (-3.611, -67.2473) construction
  line L470 (-3.611, -67.2473) -> (-3.611, -67.4872) construction
  line L471 (-3.611, -67.4872) -> (-3.611, -70.3584)
  spline S28 degree 2 poles (-3.611, -70.3584) (-3.611, -70.5983) (-3.8509, -70.5983) knots 0 0 0 1 1 1
  line L472 (-3.611, -70.3584) -> (-3.611, -70.5983) construction
  line L473 (-3.611, -70.5983) -> (-3.8509, -70.5983) construction
  spline S29 degree 2 poles (-3.8509, -70.5983) (-4.0908, -70.5983) (-4.0908, -70.3584) knots 0 0 0 1 1 1
  line L474 (-3.8509, -70.5983) -> (-4.0908, -70.5983) construction
  line L475 (-4.0908, -70.5983) -> (-4.0908, -70.3584) construction
  spline S30 degree 2 poles (-5.5224, -70.3584) (-5.5224, -70.5983) (-5.7624, -70.5983) knots 0 0 0 1 1 1
  line L476 (-5.5224, -70.3584) -> (-5.5224, -70.5983) construction
  line L477 (-5.5224, -70.5983) -> (-5.7624, -70.5983) construction
  spline S31 degree 2 poles (-5.7624, -70.5983) (-6.0023, -70.5983) (-6.0023, -70.3584) knots 0 0 0 1 1 1
  line L478 (-5.7624, -70.5983) -> (-6.0023, -70.5983) construction
  line L479 (-6.0023, -70.5983) -> (-6.0023, -70.3584) construction
  line L480 (-6.0023, -70.3584) -> (-6.0023, -67.4872)
  spline S32 degree 2 poles (-6.0023, -67.4872) (-6.0023, -67.2473) (-5.7624, -67.2473) knots 0 0 0 1 1 1
  line L481 (-6.0023, -67.4872) -> (-6.0023, -67.2473) construction
  line L482 (-6.0023, -67.2473) -> (-5.7624, -67.2473) construction
  spline S33 degree 2 poles (-5.7624, -67.2473) (-5.5224, -67.2473) (-5.5224, -67.4872) knots 0 0 0 1 1 1
  line L483 (-5.7624, -67.2473) -> (-5.5224, -67.2473) construction
  line L484 (-5.5224, -67.2473) -> (-5.5224, -67.4872) construction
  spline S34 degree 2 poles (-8.0137, -70.1185) (-7.7818, -70.1185) (-7.4419, -69.7826) (-7.4419, -69.5426) knots 0 0 0 1 2 2 2
  line L485 (-8.0137, -70.1185) -> (-7.7818, -70.1185) construction
  line L486 (-7.7818, -70.1185) -> (-7.4419, -69.7826) construction
  line L487 (-7.4419, -69.7826) -> (-7.4419, -69.5426) construction
  line L488 (-7.4419, -69.5426) -> (-7.4419, -68.303)
  spline S35 degree 2 poles (-7.4419, -68.303) (-7.4419, -68.0671) (-7.7818, -67.7272) (-8.0137, -67.7272) knots 0 0 0 1 2 2 2
  line L489 (-7.4419, -68.303) -> (-7.4419, -68.0671) construction
  line L490 (-7.4419, -68.0671) -> (-7.7818, -67.7272) construction
  line L491 (-7.7818, -67.7272) -> (-8.0137, -67.7272) construction
  line L492 (-8.0137, -67.7272) -> (-8.3016, -67.7272)
  spline S36 degree 2 poles (-8.3016, -67.7272) (-8.5376, -67.7272) (-8.8735, -68.0671) (-8.8735, -68.303) knots 0 0 0 1 2 2 2
  line L493 (-8.3016, -67.7272) -> (-8.5376, -67.7272) construction
  line L494 (-8.5376, -67.7272) -> (-8.8735, -68.0671) construction
  line L495 (-8.8735, -68.0671) -> (-8.8735, -68.303) construction
  line L496 (-8.8735, -68.303) -> (-8.8735, -69.5426)
  spline S37 degree 2 poles (-8.8735, -69.5426) (-8.8735, -69.7826) (-8.5376, -70.1185) (-8.3016, -70.1185) knots 0 0 0 1 2 2 2
  line L497 (-8.8735, -69.5426) -> (-8.8735, -69.7826) construction
  line L498 (-8.8735, -69.7826) -> (-8.5376, -70.1185) construction
  line L499 (-8.5376, -70.1185) -> (-8.3016, -70.1185) construction
  line L500 (-8.3016, -70.1185) -> (-8.0137, -70.1185)
  line L501 (-8.0137, -70.5983) -> (-8.3016, -70.5983)
  spline S38 degree 2 poles (-8.3016, -70.5983) (-8.7335, -70.5983) (-9.3533, -69.9825) (-9.3533, -69.5466) knots 0 0 0 1 2 2 2
  line L502 (-8.3016, -70.5983) -> (-8.7335, -70.5983) construction
  line L503 (-8.7335, -70.5983) -> (-9.3533, -69.9825) construction
  line L504 (-9.3533, -69.9825) -> (-9.3533, -69.5466) construction
  line L505 (-9.3533, -69.5466) -> (-9.3533, -68.299)
  spline S39 degree 2 poles (-9.3533, -68.299) (-9.3533, -67.8631) (-8.7335, -67.2473) (-8.3016, -67.2473) knots 0 0 0 1 2 2 2
  line L506 (-9.3533, -68.299) -> (-9.3533, -67.8631) construction
  line L507 (-9.3533, -67.8631) -> (-8.7335, -67.2473) construction
  line L508 (-8.7335, -67.2473) -> (-8.3016, -67.2473) construction
  line L509 (-8.3016, -67.2473) -> (-8.0137, -67.2473)
  spline S40 degree 2 poles (-8.0137, -67.2473) (-7.5778, -67.2473) (-6.962, -67.8631) (-6.962, -68.299) knots 0 0 0 1 2 2 2
  line L510 (-8.0137, -67.2473) -> (-7.5778, -67.2473) construction
  line L511 (-7.5778, -67.2473) -> (-6.962, -67.8631) construction
  line L512 (-6.962, -67.8631) -> (-6.962, -68.299) construction
  line L513 (-6.962, -68.299) -> (-6.962, -69.5466)
  spline S41 degree 2 poles (-6.962, -69.5466) (-6.962, -69.9865) (-7.5778, -70.5983) (-8.0137, -70.5983) knots 0 0 0 1 2 2 2
  line L514 (-6.962, -69.5466) -> (-6.962, -69.9865) construction
  line L515 (-6.962, -69.9865) -> (-7.5778, -70.5983) construction
  line L516 (-7.5778, -70.5983) -> (-8.0137, -70.5983) construction
  line L517 (-15.6236, -69.5946) -> (-15.6236, -70.3584)
  spline S42 degree 2 poles (-15.6236, -70.3584) (-15.6236, -70.5983) (-15.8635, -70.5983) knots 0 0 0 1 1 1
  line L518 (-15.6236, -70.3584) -> (-15.6236, -70.5983) construction
  line L519 (-15.6236, -70.5983) -> (-15.8635, -70.5983) construction
  spline S43 degree 2 poles (-15.8635, -70.5983) (-16.1034, -70.5983) (-16.1034, -70.3584) knots 0 0 0 1 1 1
  line L520 (-15.8635, -70.5983) -> (-16.1034, -70.5983) construction
  line L521 (-16.1034, -70.5983) -> (-16.1034, -70.3584) construction
  line L522 (-16.1034, -70.3584) -> (-16.1034, -67.4872)
  spline S44 degree 2 poles (-16.1034, -67.4872) (-16.1034, -67.2473) (-15.8635, -67.2473) knots 0 0 0 1 1 1
  line L523 (-16.1034, -67.4872) -> (-16.1034, -67.2473) construction
  line L524 (-16.1034, -67.2473) -> (-15.8635, -67.2473) construction
  spline S45 degree 2 poles (-15.8635, -67.2473) (-15.6236, -67.2473) (-15.6236, -67.4872) knots 0 0 0 1 1 1
  line L525 (-15.8635, -67.2473) -> (-15.6236, -67.2473) construction
  line L526 (-15.6236, -67.2473) -> (-15.6236, -67.4872) construction
  spline S46 degree 2 poles (-14.104, -67.3033) (-14.04, -67.2313) (-13.952, -67.2313) knots 0 0 0 1 1 1
  line L527 (-14.104, -67.3033) -> (-14.04, -67.2313) construction
  line L528 (-14.04, -67.2313) -> (-13.952, -67.2313) construction
  spline S47 degree 2 poles (-13.952, -67.2313) (-13.8561, -67.2313) (-13.7121, -67.3873) (-13.7121, -67.4912) knots 0 0 0 1 2 2 2
  line L529 (-13.952, -67.2313) -> (-13.8561, -67.2313) construction
  line L530 (-13.8561, -67.2313) -> (-13.7121, -67.3873) construction
  line L531 (-13.7121, -67.3873) -> (-13.7121, -67.4912) construction
  spline S48 degree 2 poles (-13.7121, -67.4912) (-13.7121, -67.5912) (-13.7881, -67.6672) knots 0 0 0 1 1 1
  line L532 (-13.7121, -67.4912) -> (-13.7121, -67.5912) construction
  line L533 (-13.7121, -67.5912) -> (-13.7881, -67.6672) construction
  spline S49 degree 2 poles (-13.7641, -70.2025) (-13.7121, -70.2824) (-13.7121, -70.3624) knots 0 0 0 1 1 1
  line L534 (-13.7641, -70.2025) -> (-13.7121, -70.2824) construction
  line L535 (-13.7121, -70.2824) -> (-13.7121, -70.3624) construction
  spline S50 degree 2 poles (-13.7121, -70.3624) (-13.7121, -70.4624) (-13.8681, -70.6063) (-13.956, -70.6063) knots 0 0 0 1 2 2 2
  line L536 (-13.7121, -70.3624) -> (-13.7121, -70.4624) construction
  line L537 (-13.7121, -70.4624) -> (-13.8681, -70.6063) construction
  line L538 (-13.8681, -70.6063) -> (-13.956, -70.6063) construction
  spline S51 degree 2 poles (-13.956, -70.6063) (-14.068, -70.6063) (-14.128, -70.5104) knots 0 0 0 1 1 1
  line L539 (-13.956, -70.6063) -> (-14.068, -70.6063) construction
  line L540 (-14.068, -70.6063) -> (-14.128, -70.5104) construction
  line L541 (-14.128, -70.5104) -> (-15.0877, -69.0308)
  spline S52 degree 2 poles (-15.0877, -69.0308) (-15.2317, -69.1827) (-15.6236, -69.5946) knots 0 0 0 1 1 1
  line L542 (-15.0877, -69.0308) -> (-15.2317, -69.1827) construction
  line L543 (-15.2317, -69.1827) -> (-15.6236, -69.5946) construction
  spline S53 degree 2 poles (-17.9709, -70.1185) (-17.775, -70.1185) (-17.4951, -69.8346) (-17.4951, -69.6386) knots 0 0 0 1 2 2 2
  line L544 (-17.9709, -70.1185) -> (-17.775, -70.1185) construction
  line L545 (-17.775, -70.1185) -> (-17.4951, -69.8346) construction
  line L546 (-17.4951, -69.8346) -> (-17.4951, -69.6386) construction
  spline S54 degree 2 poles (-18.4508, -67.7272) (-18.6467, -67.7272) (-18.9266, -68.0111) (-18.9266, -68.207) knots 0 0 0 1 2 2 2
  line L547 (-18.4508, -67.7272) -> (-18.6467, -67.7272) construction
  line L548 (-18.6467, -67.7272) -> (-18.9266, -68.0111) construction
  line L549 (-18.9266, -68.0111) -> (-18.9266, -68.207) construction
  line L550 (-18.9266, -68.207) -> (-18.9266, -69.6386)
  spline S55 degree 2 poles (-18.9266, -69.6386) (-18.9266, -69.8346) (-18.6467, -70.1185) (-18.4508, -70.1185) knots 0 0 0 1 2 2 2
  line L551 (-18.9266, -69.6386) -> (-18.9266, -69.8346) construction
  line L552 (-18.9266, -69.8346) -> (-18.6467, -70.1185) construction
  line L553 (-18.6467, -70.1185) -> (-18.4508, -70.1185) construction
  line L554 (-18.4508, -70.1185) -> (-17.9709, -70.1185)
  line L555 (-17.9709, -70.5983) -> (-18.4508, -70.5983)
  spline S56 degree 2 poles (-18.4508, -70.5983) (-18.8427, -70.5983) (-19.4065, -70.0385) (-19.4065, -69.6426) knots 0 0 0 1 2 2 2
  line L556 (-18.4508, -70.5983) -> (-18.8427, -70.5983) construction
  line L557 (-18.8427, -70.5983) -> (-19.4065, -70.0385) construction
  line L558 (-19.4065, -70.0385) -> (-19.4065, -69.6426) construction
  line L559 (-19.4065, -69.6426) -> (-19.4065, -68.203)
  spline S57 degree 2 poles (-19.4065, -68.203) (-19.4065, -67.8071) (-18.8427, -67.2473) (-18.4508, -67.2473) knots 0 0 0 1 2 2 2
  line L560 (-19.4065, -68.203) -> (-19.4065, -67.8071) construction
  line L561 (-19.4065, -67.8071) -> (-18.8427, -67.2473) construction
  line L562 (-18.8427, -67.2473) -> (-18.4508, -67.2473) construction
  line L563 (-18.4508, -67.2473) -> (-17.2551, -67.2473)
  spline S58 degree 2 poles (-17.2551, -67.2473) (-17.0152, -67.2473) (-17.0152, -67.4872) knots 0 0 0 1 1 1
  line L564 (-17.2551, -67.2473) -> (-17.0152, -67.2473) construction
  line L565 (-17.0152, -67.2473) -> (-17.0152, -67.4872) construction
  line L566 (-17.0152, -67.4872) -> (-17.0152, -69.6346)
  spline S59 degree 2 poles (-17.0152, -69.6346) (-17.0152, -69.9945) (-16.6793, -70.1385) knots 0 0 0 1 1 1
  line L567 (-17.0152, -69.6346) -> (-17.0152, -69.9945) construction
  line L568 (-17.0152, -69.9945) -> (-16.6793, -70.1385) construction
  spline S60 degree 2 poles (-16.6793, -70.1385) (-16.5313, -70.1985) (-16.5313, -70.3504) knots 0 0 0 1 1 1
  line L569 (-16.6793, -70.1385) -> (-16.5313, -70.1985) construction
  line L570 (-16.5313, -70.1985) -> (-16.5313, -70.3504) construction
  spline S61 degree 2 poles (-16.5313, -70.3504) (-16.5313, -70.4504) (-16.6673, -70.6023) (-16.7673, -70.6023) knots 0 0 0 1 2 2 2
  line L571 (-16.5313, -70.3504) -> (-16.5313, -70.4504) construction
  line L572 (-16.5313, -70.4504) -> (-16.6673, -70.6023) construction
  line L573 (-16.6673, -70.6023) -> (-16.7673, -70.6023) construction
  spline S62 degree 2 poles (-16.7673, -70.6023) (-16.8192, -70.6023) (-16.8712, -70.5784) knots 0 0 0 1 1 1
  line L574 (-16.7673, -70.6023) -> (-16.8192, -70.6023) construction
  line L575 (-16.8192, -70.6023) -> (-16.8712, -70.5784) construction
  spline S63 degree 2 poles (-16.8712, -70.5784) (-17.1112, -70.4744) (-17.2591, -70.2824) knots 0 0 0 1 1 1
  line L576 (-16.8712, -70.5784) -> (-17.1112, -70.4744) construction
  line L577 (-17.1112, -70.4744) -> (-17.2591, -70.2824) construction
  spline S64 degree 2 poles (-17.2591, -70.2824) (-17.547, -70.5983) (-17.9709, -70.5983) knots 0 0 0 1 1 1
  line L578 (-17.2591, -70.2824) -> (-17.547, -70.5983) construction
  line L579 (-17.547, -70.5983) -> (-17.9709, -70.5983) construction
  spline S65 degree 2 poles (-5.566, -57.1525) (-6.0458, -57.1525) (-6.0458, -56.6726) knots 0 0 0 1 1 1
  line L580 (-5.566, -57.1525) -> (-6.0458, -57.1525) construction
  line L581 (-6.0458, -57.1525) -> (-6.0458, -56.6726) construction
  spline S66 degree 2 poles (-6.0458, -56.6726) (-6.0458, -56.1927) (-5.566, -56.1927) knots 0 0 0 1 1 1
  line L582 (-6.0458, -56.6726) -> (-6.0458, -56.1927) construction
  line L583 (-6.0458, -56.1927) -> (-5.566, -56.1927) construction
  line L584 (-5.566, -56.1927) -> (-1.735, -56.1927)
  spline S67 degree 2 poles (-1.735, -56.1927) (-1.2632, -56.1927) (-1.2632, -56.6726) knots 0 0 0 1 1 1
  line L585 (-1.735, -56.1927) -> (-1.2632, -56.1927) construction
  line L586 (-1.2632, -56.1927) -> (-1.2632, -56.6726) construction
  spline S68 degree 2 poles (-1.2632, -56.6726) (-1.2632, -57.1525) (-1.735, -57.1525) knots 0 0 0 1 1 1
  line L587 (-1.2632, -56.6726) -> (-1.2632, -57.1525) construction
  line L588 (-1.2632, -57.1525) -> (-1.735, -57.1525) construction
  line L589 (-1.735, -57.1525) -> (-5.566, -57.1525)
  spline S69 degree 2 poles (-11.3963, -61.4681) (-11.5427, -61.4681) (-11.6305, -61.3315) knots 0 0 0 1 1 1
  line L590 (-11.3963, -61.4681) -> (-11.5427, -61.4681) construction
  line L591 (-11.5427, -61.4681) -> (-11.6305, -61.3315) construction
  spline S70 degree 2 poles (-13.4746, -61.3315) (-13.5624, -61.4681) (-13.7088, -61.4681) knots 0 0 0 1 1 1
  line L592 (-13.4746, -61.3315) -> (-13.5624, -61.4681) construction
  line L593 (-13.5624, -61.4681) -> (-13.7088, -61.4681) construction
  spline S71 degree 2 poles (-13.7088, -61.4681) (-13.8259, -61.4681) (-14.0162, -61.2925) (-14.0162, -61.1705) knots 0 0 0 1 2 2 2
  line L594 (-13.7088, -61.4681) -> (-13.8259, -61.4681) construction
  line L595 (-13.8259, -61.4681) -> (-14.0162, -61.2925) construction
  line L596 (-14.0162, -61.2925) -> (-14.0162, -61.1705) construction
  spline S72 degree 2 poles (-14.0162, -61.1705) (-14.0162, -61.0876) (-13.9674, -61.0047) knots 0 0 0 1 1 1
  line L597 (-14.0162, -61.1705) -> (-14.0162, -61.0876) construction
  line L598 (-14.0162, -61.0876) -> (-13.9674, -61.0047) construction
  spline S73 degree 2 poles (-13.9674, -57.8336) (-14.0162, -57.7506) (-14.0162, -57.6677) knots 0 0 0 1 1 1
  line L599 (-13.9674, -57.8336) -> (-14.0162, -57.7506) construction
  line L600 (-14.0162, -57.7506) -> (-14.0162, -57.6677) construction
  spline S74 degree 2 poles (-14.0162, -57.6677) (-14.0162, -57.5457) (-13.8259, -57.3701) (-13.7088, -57.3701) knots 0 0 0 1 2 2 2
  line L601 (-14.0162, -57.6677) -> (-14.0162, -57.5457) construction
  line L602 (-14.0162, -57.5457) -> (-13.8259, -57.3701) construction
  line L603 (-13.8259, -57.3701) -> (-13.7088, -57.3701) construction
  spline S75 degree 2 poles (-13.7088, -57.3701) (-13.5624, -57.3701) (-13.4746, -57.5067) knots 0 0 0 1 1 1
  line L604 (-13.7088, -57.3701) -> (-13.5624, -57.3701) construction
  line L605 (-13.5624, -57.3701) -> (-13.4746, -57.5067) construction
  spline S76 degree 2 poles (-11.6305, -57.5067) (-11.5427, -57.3701) (-11.3963, -57.3701) knots 0 0 0 1 1 1
  line L606 (-11.6305, -57.5067) -> (-11.5427, -57.3701) construction